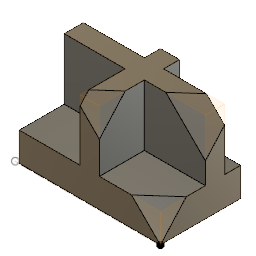
Task2a v0 (Autodesk Fusion 360 design; units mm, degrees)
Autodesk Fusion 360 part; units mm, degrees
sketch "Sketch1" plane through (0, 0, 0) normal (0, 1, 0) x (1, 0, 0)
  line L0 (0, 0) -> (0, 50)
  line L1 (0, 50) -> (88, 50)
  line L2 (88, 50) -> (88, 0)
  line L3 (88, 0) -> (0, 0)
  dimension "d1" = 50
  dimension "d2" = 88
  constraint coincident L0.start L3.end
  constraint vertical L0
  constraint perpendicular L0 L1
  constraint perpendicular L1 L2
  constraint perpendicular L0 L3
  measures "d1" distance of L0.start L0.end
  measures "d2" distance of L0.end L1.end
extrude "Extrude1" add sketch "Sketch1" along normal blind 18
sketch "Sketch2" plane through (0, 18, 0) normal (0, 1, 0) x (-1, 0, 0)
  line L0 (-88, 0) -> (-88, -50)
  line L1 (-88, -50) -> (0, -50)
  line L2 (0, -50) -> (0, 0)
  line L3 (0, 0) -> (-88, 0)
  line L4 (-38, 0) -> (-38, -28)
  line L5 (-38, -28) -> (0, -28)
  line L6 (0, -28) -> (0, -40)
  line L7 (0, -40) -> (-38, -40)
  line L8 (-38, -40) -> (-38, -50)
  line L9 (-38, -50) -> (-50, -50)
  line L10 (-50, -50) -> (-50, -40)
  line L11 (-50, -40) -> (-88, -40)
  line L12 (-88, -40) -> (-88, -28)
  line L13 (-50, -28) -> (-50, 0)
  line L14 (-38, 0) -> (-50, 0)
  line L15 (-50, -28) -> (-88, -28)
  line L16 (-50, 0) -> (-38, 0)
  constraint coincident L3 L4.start
  constraint perpendicular L2 L5
  constraint coincident L2 L6.end
  constraint perpendicular L6 L7
  constraint coincident L1 L8.end
  constraint perpendicular L1 L8
  constraint perpendicular L8 L9
  constraint perpendicular L1 L10
  constraint coincident L0 L11.end
  constraint perpendicular L0 L11
  constraint coincident L0 L12.end
  constraint coincident L3 L13.end
  constraint perpendicular L3 L13
  constraint perpendicular L12 L15
extrude "Extrude2" add sketch "Sketch2" along normal blind 38 contours L0 L1 L2 L3 L4 L5 L6 L7 L8 L9 L10 L11 L12 L13 L14 L15 L16
sketch "Sketch3" plane through (0, 0, 0) normal (0, 0, 1) x (1, 0, 0)
sketch "Sketch4" plane through (0, 0, 0) normal (0, 0, 1) x (1, 0, 0)
  line L0 (0, 0) -> (88, 0)
  line L1 (88, 0) -> (88, 18)
  line L2 (88, 18) -> (50, 18)
  line L3 (50, 18) -> (50, 56)
  line L4 (50, 56) -> (38, 56)
  line L5 (38, 56) -> (38, 18)
  line L6 (38, 18) -> (0, 18)
  line L7 (0, 18) -> (0, 0)
  line L8 (88, 0) -> (-2.3828, 0) construction
  constraint horizontal L8
  constraint coincident L0.end L1.start
sketch "Sketch5" plane through (88, 0, 0) normal (1, 0, 0) x (0, 0, -1)
  line L0 (0, 0) -> (50, 0)
  line L1 (50, 0) -> (50, 18)
  line L2 (50, 18) -> (40, 18)
  line L3 (40, 18) -> (40, 56)
  line L4 (40, 56) -> (28, 56)
  line L5 (28, 56) -> (28, 18)
  line L6 (28, 18) -> (0, 18)
  line L7 (0, 18) -> (0, 0)
sketch "Sketch6" plane through (0, 0, 0) normal (0, 0, 1) x (1, 0, 0)
sketch "Sketch7" plane through (0, 0, 0) normal (0, 0, 1) x (1, 0, 0)
sketch "Sketch9" plane through (0, 0, 0) normal (0, 0, 1) x (1, 0, 0)
sketch "Sketch10" plane through (0, 56, 0) normal (0, 1, 0) x (-1, 0, 0)
  line L0 (-50, -28) -> (-88, -28)
  line L1 (-88, -28) -> (-88, -40)
  line L2 (-88, -40) -> (-50, -40)
  line L3 (-50, -40) -> (-50, -50)
  line L4 (-50, -50) -> (-38, -50)
  line L5 (-38, -50) -> (-38, -40)
  line L6 (-38, -40) -> (0, -40)
  line L7 (0, -40) -> (0, -28)
  line L8 (0, -28) -> (-38, -28)
  line L9 (-38, -28) -> (-38, 0)
  line L10 (-38, 0) -> (-50, 0)
  line L11 (-50, 0) -> (-50, -28)
sketch "Sketch11" plane through (0, 0, 0) normal (0, 0, 1) x (1, 0, 0)
ref_plane "WorkPlane1" through (88, 0, 0) normal (-0.554325, -0.554325, -0.620844) x (0.707107, -0.707107, 0)
sketch "Sketch12" plane through (88, 0, 0) normal (-0.554325, -0.554325, -0.620844) x (0.707107, -0.707107, 0)
  line L0 (-83.6898, 2.465) -> (-36.8291, -71.3922)
  line L1 (-36.8291, -71.3922) -> (9.1129, 2.465)
  line L2 (9.1129, 2.465) -> (-83.6898, 2.465)
  constraint horizontal L2
extrude "Extrude3" cut sketch "Sketch12" against normal blind 15
